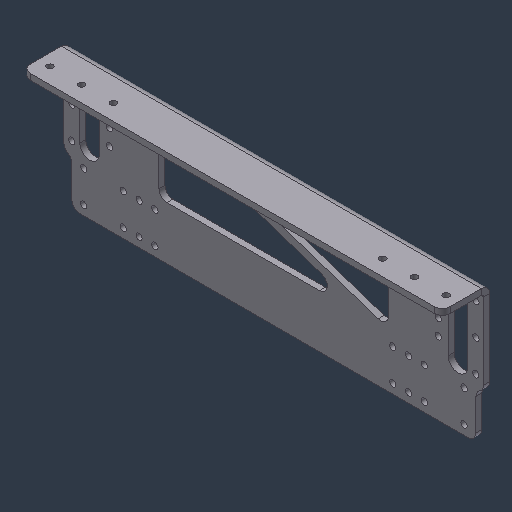
# Autodesk Inventor part: PLATE,MOUNT,DRIVE,ELEVATOR
Saved by Autodesk Inventor 2024.3 (Build 283343000, 343)
## iProperties
Category: _
Manager: _
Created: 2025-01-29
Part Number: PLATE,MOUNT,DRIVE,ELEVATOR
Checked By: 00
Engr Approved By: _
User Status: Work In Process
Material: Sheet Metal, Aluminum, 3003
Description: SHEET METAL (mm)
Document SubType Name: Sheet Metal
Mfg Approved By: John.Thibert
Designer: John.Thibert
Manufacturer: Standard
Standards Organization: Custom
Density: 2.73 g/cm^3
Sheet Metal Rule: Default
Appearance: Metal-AL-6061 (Flat)
Mass: 466.588 g
Surface Area: 833.226 cm^2
Volume: 170.911 cm^3
Flat Pattern Width: 14.1707 cm
Flat Pattern Length: 33.655 cm
Flat Pattern Area: 476.917 cm^2
Sheet Metal Width: 5.579 in
Sheet Metal Length: 13.250 in
Sheet Metal Area: 73.922 in^2
ILogicPurgeVersion: 2.2.20.20
OnSaveVersion: 3.5.0.0
OnSaveAssembly: COREAutomationManager
CN_MASS: 0.47
CL_runCount: 1
CN_SERVICEABLE: _
FIRST_DESCRIPTION: _
SECOND_DESCRIPTION: _
THIRD_DESCRIPTION: _
ModelCat: Uncategorized
MaterialName: Sheet Metal, Aluminum, 3003
Subject: _
Author: John.Thibert
Keywords: -
Revision Number: A
Autodesk Inventor part; units mm, degrees
ref_plane "YZ Plane" through (0, 0, 0) normal (1, 0, 0) x (0, 1, 0)
ref_plane "XZ Plane" through (0, 0, 0) normal (0, 1, 0) x (-1, 0, 0)
ref_plane "XY Plane" through (0, 0, 0) normal (0, 0, 1) x (1, 0, 0)
sketch "Sketch1" plane through (0, 0, 0) normal (0, 0, 1) x (1, 0, 0)
  line L0 (168.275, -51.9684) -> (-168.275, -51.9684)
  line L1 (-168.275, -51.9684) -> (-168.275, 51.9684)
  line L2 (-168.275, 51.9684) -> (168.275, 51.9684)
  line L3 (168.275, 51.9684) -> (168.275, -51.9684)
  line L4 (168.275, -51.9684) -> (-168.275, 51.9684) construction
  line L5 (-168.275, -51.9684) -> (168.275, 51.9684) construction
  point P0 (0, 0)
  dimension "d0" = 336.55
  dimension "d1" = 103.9368
  measures "d0" distance of L1.end L2.end
  measures "d1" distance of L0.end L1.end
extrude "Plate1" add sketch "Sketch1" along normal mid plane 4.7625
sketch "Sketch2" plane through (-168.275, 53.9684, 4.3812) normal (0, 1, 0) x (-1, 0, 0)
  line L0 (-336.55, 0) -> (0, 0)
  line L1 (0, 0) -> (0, 31.3375)
  line L2 (0, 31.3375) -> (-336.55, 31.3375)
  line L3 (-336.55, 31.3375) -> (-336.55, 0)
  constraints: 6 end point, 1 horizontal, 1 perpendicular, 1 vertical
edge flange "Flange1" height 38.1 angle 90 thickness 4.7625 bend radius 2 thickness toward (0, 1, 0) relief straight relief width 4.7625 relief depth 2.3813 edges at (0, 51.9684, 2.3813) wall of the first edge with corners at (168.275, 53.9684, 4.3812) (-168.275, 53.9684, 4.3812) (-168.275, 53.9684, 35.7188) (168.275, 53.9684, 35.7188)
bend "Bend1"
corner "Corner1"
sketch "Sketch3" plane through (0, 0, 2.3813) normal (0, 0, 1) x (1, 0, 0)
  line L0 (161.925, -4.7691) -> (-161.925, -4.7691) construction
  line L1 (-161.925, -4.7691) -> (-161.925, 46.0309) construction
  line L2 (-161.925, 46.0309) -> (161.925, 46.0309) construction
  line L3 (161.925, 46.0309) -> (161.925, -4.7691) construction
  line L4 (161.925, -4.7691) -> (-161.925, 46.0309) construction
  line L5 (-161.925, -4.7691) -> (161.925, 46.0309) construction
  line L6 (-235.585, 0) -> (235.585, 0) construction
  line L7 (0, 79.4687) -> (0, -73.8746) construction
  line L8 (168.275, 58.7309) -> (-168.275, 58.7309) construction
  point P0 (0, 20.6309)
  point P1 (-161.925, 20.6309)
  point P2 (161.925, 20.6309)
  dimension "d13" = 323.85
  dimension "d14" = 50.8
  dimension "d44" = 12.7
  constraints: 12 end point, 4 coincident, 4 midpoint, 2 parallel, 1 horizontal, 1 perpendicular, 1 point on line
  measures "d13" distance of L1.end L2.end
  measures "d14" distance of L0.end L1.end
  measures "d44" distance between parallel lines of L2 L8
hole "Hole1" at (-161.925, 46.0309, 2.3813) at (161.925, 46.0309, 2.3813) at (-161.925, 20.6309, 2.3813) at (-161.925, -4.7691, 2.3813) at (161.925, 20.6309, 2.3813) at (161.925, -4.7691, 2.3813) direction (0, 0, -1) diameter 5.1054 end through all start extended yes clearance for "Flat Head Machine Screw (82)" size "#10" standard "Ansi Unified Screw Threads"
sketch "Sketch4" plane through (0, 0, 2.3813) normal (0, 0, 1) x (1, 0, 0)
  line L0 (95.25, -12.7066) -> (-95.25, -12.7066) construction
  line L1 (-95.25, -12.7066) -> (-95.25, 50.7934) construction
  line L2 (-95.25, 50.7934) -> (95.25, 50.7934) construction
  line L3 (95.25, 50.7934) -> (95.25, -12.7066) construction
  line L4 (95.25, -12.7066) -> (-95.25, 50.7934) construction
  line L5 (-95.25, -12.7066) -> (95.25, 50.7934) construction
  line L6 (-75.6848, 47.6184) -> (92.075, 47.6184)
  line L7 (92.075, 47.6184) -> (92.075, -8.3015)
  line L8 (92.075, -8.3015) -> (-75.6848, 47.6184)
  line L9 (-92.075, -9.5316) -> (75.6848, -9.5316)
  line L10 (75.6848, -9.5316) -> (-92.075, 46.3883)
  line L11 (-92.075, 46.3883) -> (-92.075, -9.5316)
  line L12 (-147.6375, -3.1816) -> (-147.6375, 41.2684) construction
  line L13 (-155.575, -3.1816) -> (-155.575, 41.2684)
  line L14 (-139.7, 41.2684) -> (-139.7, -3.1816)
  arc A0 (-155.575, -3.1816) -> (-139.7, -3.1816) centre (-147.6375, -3.1816) ccw
  arc A1 (-139.7, 41.2684) -> (-155.575, 41.2684) centre (-147.6375, 41.2684) ccw
  line L15 (0, 79.4687) -> (0, -73.8746) construction
  line L16 (147.6375, -3.1816) -> (147.6375, 41.2684) construction
  line L17 (155.575, -3.1816) -> (155.575, 41.2684)
  line L18 (139.7, 41.2684) -> (139.7, -3.1816)
  arc A2 (139.7, -3.1816) -> (155.575, -3.1816) centre (147.6375, -3.1816) ccw
  arc A3 (155.575, 41.2684) -> (139.7, 41.2684) centre (147.6375, 41.2684) ccw
  line L19 (-147.6375, 19.0434) -> (147.6375, 19.0434) construction
  line L20 (-235.585, 0) -> (235.585, 0) construction
  line L21 (168.275, 58.7309) -> (-168.275, 58.7309) construction
  line L22 (-168.275, -13.8684) -> (-161.925, -13.8684)
  line L23 (-161.925, -13.8684) -> (-161.925, -51.9684)
  line L24 (168.275, -51.9684) -> (-168.275, -51.9684) projected
  line L25 (-168.275, -51.9684) -> (-168.275, 51.9684) projected
  line L26 (168.275, 51.9684) -> (168.275, -51.9684) projected
  line L27 (161.925, -51.9684) -> (161.925, -13.8684)
  line L28 (161.925, -13.8684) -> (168.275, -13.8684)
  point P0 (0, 19.0434)
  dimension "d22" = 63.5
  dimension "d23" = 190.5
  dimension "d24" = 3.175
  dimension "d25" = 3.175
  dimension "d29" = 7.9375
  dimension "d30" = 44.45
  dimension "d31" = 147.6375
  dimension "d45" = 39.6875
  dimension "d85" = 38.1
  dimension "d86" = 6.35
  constraints: 50 end point, 8 point on circle, 7 symmetric about line, 6 perpendicular, 4 centre point, 4 midpoint, 4 point on line, 4 tangent, 3 parallel, 2 equal length, 2 horizontal, 2 vertical, 1 horizontal alignment, 6 other
  measures "d22" distance of L0.end L1.end
  measures "d23" distance of L1.end L2.end
  measures "d24" distance between parallel lines of L0 L9
  measures "d25" distance between parallel lines of L2 L6
  measures "d29" radius of A1
  measures "d30" distance of L12.start L12.end
  measures "d31" distance between parallel lines of L12 L15
  measures "d45" distance between parallel lines of L19 L21
  measures "d85" distance of L22.end L23.end
  measures "d86" distance of L22.start L22.end
extrude "Cut1" cut sketch "Sketch4" against normal through all
sketch "Sketch6" plane through (0, 0, 2.3813) normal (0, 0, 1) x (1, 0, 0)
  line L0 (-120.65, -19.05) -> (-120.65, -44.45) construction
  line L1 (-168.275, -51.9684) -> (-168.275, 51.9684) construction
  point P0 (0, 0)
  dimension "d46" = 25.4
  dimension "d47" = 47.625
  dimension "d58" = 19.05
  constraints: 2 coincident, 2 end point, 1 vertical
  measures "d46" distance of L0.start L0.end
  measures "d47" distance between parallel lines of L1 L0
  measures "d58" vertical distance of point (-120.65, -19.05) point (0, 0)
hole "Hole2" at (-120.65, -19.05, 2.3813) at (-120.65, -44.45, 2.3813) direction (0, 0, -1) diameter 5.1054 end through all clearance for "Flat Head Machine Screw (82)" size "#10" standard "Ansi Unified Screw Threads"
pattern_linear "Rectangular Pattern1" count 2 spacing 31.75 along (-1, 0, 0) of "Hole2"
pattern_linear "Rectangular Pattern2" count 3 spacing 12.7 along (1, 0, 0) of "Hole2"
sketch "Sketch7" plane through (0, 0, 2.3813) normal (0, 0, 1) x (1, 0, 0)
  line L0 (-139.7, 41.2684) -> (-139.7, -3.1816) construction
  line L1 (-131.7625, 31.8516) -> (-131.7625, 6.4516) construction
  point P0 (0, 0)
  point P1 (-131.7625, 19.1516)
  dimension "d62" = 25.4
  dimension "d63" = 7.9375
  dimension "d64" = 19.1516
  constraints: 2 coincident, 2 end point, 1 midpoint, 1 vertical
  measures "d62" distance of L1.start L1.end
  measures "d63" distance between parallel lines of L0 L1
  measures "d64" vertical distance of point (0, 0) point (-131.763, 19.152)
hole "Hole3" at (-131.7625, 31.8516, 2.3813) at (-131.7625, 19.1516, 2.3813) at (-131.7625, 6.4516, 2.3813) direction (0, 0, -1) diameter 5.1054 end through all clearance for "Flat Head Machine Screw (82)" size "#10" standard "Ansi Unified Screw Threads"
sketch "Sketch8" plane through (-168.275, 53.9684, 4.3812) normal (0, -1, 0) x (1, 0, 0)
  line L0 (0, -2) -> (336.55, -2) construction
  line L1 (0, 31.3375) -> (0, 0) construction
  point P0 (168.275, -4.3813)
  point P1 (9.525, 18.6375)
  dimension "d72" = 20.6375
  dimension "d73" = 9.525
  measures "d72" distance from line of point (9.525, 18.638) L0
  measures "d73" distance from line of point (9.525, 18.638) L1
mirror "Mirror1" about plane through (0, 0, 0) normal (1, 0, 0) of "Hole2", "Rectangular Pattern1", "Rectangular Pattern2", "Hole3"
hole "Hole4" at (-158.75, 53.9684, 23.0187) direction (0, 1, 0) diameter 5.1054 depth 4.7625 tip angle 118 clearance for "Flat Head Machine Screw (82)" size "#10" standard "Ansi Unified Screw Threads"
pattern_linear "Rectangular Pattern3" count 3 spacing 25.4 along (1, 0, 0) of "Hole4"
mirror "Mirror2" about plane through (0, 0, 0) normal (1, 0, 0) of "Hole4", "Rectangular Pattern3"
fillet "Corner Round3" radius 6.35 8 edges at (-92.075, -9.5316, 0) (75.6848, -9.5316, 0) (-92.075, 46.3883, 0) (161.925, -13.8684, 0) (-161.925, -13.8684, 0) (92.075, -8.3015, 0) (-75.6848, 47.6184, 0) (92.075, 47.6184, 0)
fillet "Corner Round3" radius 6.35 2 edges at (-168.275, 56.3496, 35.7188) (168.275, 56.3497, 35.7188)
fillet "Corner Round3" radius 6.35 4 edges at (-168.275, -13.8684, 0) (-161.925, -51.9684, 0) (168.275, -13.8684, 0) (161.925, -51.9684, 0)
equation "\"d20\" = Thickness"
equation "\"d25\" = d24"
equation "\"d26\" = Thickness"
equation "\"d70\" = Thickness"
equation "\"d79\" = Thickness"
equation "\"d2\" = Thickness"
equation "\"d3\" = BendReliefWidth"
equation "\"d4\" = BendReliefDepth"
equation "\"d5\" = MinimumRemnant"
equation "\"d6\" = TransitionRadius"
equation "\"d10\" = CornerReliefSize"
equation "\"d11\" = GapSize"
equation "\"d12\" = JacobiRadiusSize"
equation "\"BendRadius\" = 1.5 * Thickness"
equation "\"BendReliefWidth\" = Thickness"
equation "\"BendReliefDepth\" = 0.5 * Thickness"
equation "\"CornerReliefSize\" = 4 * Thickness"
equation "\"MinimumRemnant\" = 2 * Thickness"
equation "\"TransitionRadius\" = BendRadius"
equation "\"JacobiRadiusSize\" = BendRadius"
equation "\"GapSize\" = Thickness"
equation "\"Thickness\" = 4.7625"
body "Solid1"
